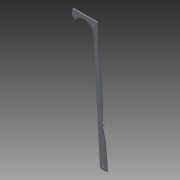
# Autodesk Inventor part: PassiveHooks3
Saved by Autodesk Inventor 2013 (Build 170138000, 138)
## iProperties
Created: 2013-02-07
Part Number: PassiveHooks3
Material: Generic
Document SubType Name: Modeling
Designer: motoennies
Density: 1 g/cm^3
Author: motoennies
Autodesk Inventor part; units mm, degrees
ref_plane "YZ Plane" through (0, 0, 0) normal (1, 0, 0) x (0, 1, 0)
ref_plane "XZ Plane" through (0, 0, 0) normal (0, 1, 0) x (-1, 0, 0)
ref_plane "XY Plane" through (0, 0, 0) normal (0, 0, 1) x (1, 0, 0)
sketch "Sketch1" plane through (0, 0, 0) normal (0, 0, 1) x (1, 0, 0)
  line L0 (82.55, -393.7) -> (48.2795, -5.3201)
  line L1 (47.853, -228.6) -> (34.8698, 1.9636)
  line L2 (57.15, -393.7) -> (82.55, -393.7)
  circle A0 centre (69.155, -381) radius 3.175
  line L3 (0, 0) -> (-58.2409, 0) construction
  line L4 (-30.2459, 17.4625) -> (-41.2445, 23.8125)
  line L5 (47.5493, 47.625) -> (47.5493, 2.9548)
  arc A1 (34.8698, 1.9636) -> (-30.2459, 17.4625) centre (0, 0) ccw
  line L6 (-41.2445, 47.625) -> (-41.2445, 23.8125)
  line L7 (-41.2445, 47.625) -> (161.9555, 47.625) construction
  line L8 (-41.2445, 47.625) -> (161.9555, 47.625) construction
  line L9 (-41.2445, 47.625) -> (161.9555, 47.625) construction
  line L10 (-41.2445, 47.625) -> (161.9555, 47.625) construction
  line L11 (-41.2445, 47.625) -> (47.5493, 47.625)
  line L12 (47.853, -228.6) -> (57.15, -393.7)
  circle A2 centre (64.77, -255.905) radius 2.3813
  circle A3 centre (34.8493, 34.925) radius 3.175
  circle A4 centre (64.77, -255.905) radius 5.5993
  line L13 (64.7552, -250.3058) -> (65.4147, -199.51)
  line L14 (63.8836, -261.4336) -> (75.2478, -310.9462)
  line L15 (75.2478, -310.9462) -> (65.4147, -199.51)
  line L16 (48.2795, -5.3201) -> (47.5493, 2.9548)
  point P0 (47.5493, 25.2899)
  point P1 (51.4288, -292.1)
  point P2 (66.5391, -212.2523)
  point P3 (73.9365, -296.0849)
  dimension "d0" = 69.85
  dimension "d1" = 30
  dimension "d2" = 57.15
  dimension "d3" = 25.4
  dimension "d4" = 393.7
  dimension "d5" = 6.35
  dimension "d6" = 12.7
  dimension "d7" = 12.7
  dimension "d8" = 4.7625
  dimension "d9" = 7.62
  dimension "d10" = 137.795
  dimension "d11" = 6.35
  dimension "d12" = 12.7
  dimension "d13" = 12.7
  dimension "d23" = 50.8
  dimension "d24" = 50.8
  constraints: 34 end point, 6 point on line, 5 centre point, 4 horizontal, 4 point on circle, 3 coincident, 2 collinear, 2 midpoint, 2 perpendicular, 2 tangent, 1 parallel, 1 vertical, 4 other
  measures "d0" diameter of A1
  measures "d1" angle of L4 L3
  measures "d2" horizontal distance of L2.start point (0, 0)
  measures "d3" distance of L0.start L2.start
  measures "d4" distance from line of point (0, 0) L2
  measures "d5" diameter of A0
  measures "d6" distance from line of L2 A0.centre
  measures "d7" distance from line of L1 A0.centre
  measures "d8" diameter of A2
  measures "d9" horizontal distance of L2.start A2.centre
  measures "d10" distance from line of L2 A2.centre
  measures "d11" diameter of A3
  measures "d12" distance from line of L11 A3.centre
  measures "d13" horizontal distance of point (47.549, 25.29) A3.centre
  measures "d23" distance of L13.start L13.end
  measures "d24" distance of L14.start L14.end
extrude "Extrusion4" add sketch "Sketch1" along normal blind 3.175 contours L2 L12 L1 A1 L4 L6 L11 L5 L16 L0 L13 A4 L14 | A4
fillet "Fillet1" radius 3.175 6 edges at (-30.2459, 17.4625, 1.5875) (47.5493, 47.625, 1.5875) (-41.2445, 47.625, 1.5875) (82.55, -393.7, 1.5875) (57.15, -393.7, 1.5875) (-41.2445, 23.8125, 1.5875)
body "Solid4"
